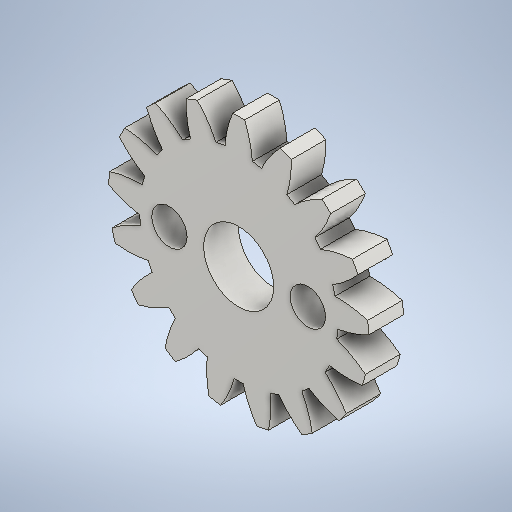
# Autodesk Inventor part: 平歯車1
Saved by Autodesk Inventor 2025.1 (Build 291241000, 241)
## iProperties
CustomPartVersion: 1
Created: 2025-05-06
Part Number: 平歯車1
Material: Steel
Document SubType Name: Modeling
Designer: yuki0520
Categories: <?xml version="1.0" encoding="UTF-16"?> <MemberInstance><Categories><FamilyTemplate><FamilyTemplateParameter ValueType="xs:double" Id="1" ObjectReferenceKey="da_z" ObjectType="kUserParameterObject"/><FamilyTemplateParameter ValueType="xs:double" Id="2" ObjectReferenceKey="da_b" ObjectType="kUserParameterObject"/><FamilyTemplateParameter ValueType="xs:double" Id="3" ObjectReferenceKey="da_beta" ObjectType="kUserParameterObject"/><FamilyTemplateParameter ValueType="xs:double" Id="4" ObjectReferenceKey="da_da" ObjectType="kUserParameterObject"/><FamilyTemplateParameter ValueType="xs:double" Id="5" ObjectReferenceKey="da_aw" ObjectType="kUserParameterObject"/><FamilyTemplateParameter ValueType="xs:string" Id="6" ObjectReferenceKey="EAIAABAAAACIAQAAAAAAAIAAAAAAAAAA" ObjectType="83910656" SubObjectId="SurfaceGeometry"/></FamilyTemplate><ParamToTemplateMap><ParamToTemplate CategoryParameter="//CategoryParameter[@InternalName='046C89C9-8512-4d59-83FE-43B91F4F132A']" TemplateParameter="1"/><ParamToTemplate CategoryParameter="//CategoryParameter[@InternalName='2552DF32-E462-4b46-AEBF-C6C7768E72AC']" TemplateParameter="2"/><ParamToTemplate CategoryParameter="//CategoryParameter[@InternalName='C9EE641D-15FC-4fae-A226-E94C4372FDD7']" TemplateParameter="3"/><ParamToTemplate><ParamToTemplate CategoryParameter="//CategoryParameter[@InternalName='00B6519A-459B-49c7-AD84-2E56D39A5744']" ConstantValue="-0.100000"/></ParamToTemplate><ParamToTemplate><ParamToTemplate CategoryParameter="//CategoryParameter[@InternalName='04B31F0E-C7A6-4894-AA32-9629BEFACF47']" ConstantValue="1.000000"/></ParamToTemplate><ParamToTemplate><ParamToTemplate CategoryParameter="//CategoryParameter[@InternalName='43CBEC2E-7847-49e7-A936-2F7889FCB2D9']" ConstantValue="0.250000"/></ParamToTemplate><ParamToTemplate><ParamToTemplate CategoryParameter="//CategoryParameter[@InternalName='B1EFC894-105D-4ebd-86BF-FA20ED196853']" ConstantValue="0.350000"/></ParamToTemplate><ParamToTemplate><ParamToTemplate CategoryParameter="//CategoryParameter[@InternalName='51175063-3D10-4879-93E8-6246FE8B403D']" ConstantValue="2060000000.000000"/></ParamToTemplate><ParamToTemplate><ParamToTemplate CategoryParameter="//CategoryParameter[@InternalName='A3A52E27-4454-46a9-B0BD-C932399B70AF']" ConstantValue="0.300000"/></ParamToTemplate><ParamToTemplate><ParamToTemplate CategoryParameter="//CategoryParameter[@InternalName='91B76062-C214-41d9-B1B9-14D2AB99603D']" ConstantValue="0.200000"/></ParamToTemplate><ParamToTemplate><ParamToTemplate CategoryParameter="//CategoryParameter[@InternalName='374E806E-8B8A-4dda-A9AA-1039D6500AD2']" ConstantValue="5.000000"/></ParamToTemplate><ParamToTemplate><ParamToTemplate CategoryParameter="//CategoryParameter[@InternalName='2D373A89-B862-43d6-8D0B-0CBF12AB9F6C']" ConstantValue="0.349066"/></ParamToTemplate><ParamToTemplate CategoryParameter="//CategoryParameter[@InternalName='37777632-D6A2-4fac-9D53-DB8ACD95C989']" TemplateParameter="4"/><ParamToTemplate CategoryParameter="//CategoryParameter[@InternalName='FD1017F1-B727-4f7e-9707-0F86F1FF9423']" TemplateParameter="5"/><ParamToTemplate><ParamToTemplate CategoryParameter="//CategoryParameter[@InternalName='9E1B4470-B2D3-4ff1-B813-535BB4CDF51A']" ConstantValue="3520000.000000"/></ParamToTemplate><ParamToTemplate><ParamToTemplate CategoryParameter="//CategoryParameter[@InternalName='F8452263-BFF6-458c-9FB1-07C4B99E95CD']" ConstantValue="11400000.000000"/></ParamToTemplate><ParamToTemplate><ParamToTemplate CategoryParameter="//CategoryParameter[@InternalName='3E3BB259-FD49-497f-8171-6EBC954A3479']" ConstantValue="2.000000"/></ParamToTemplate><ParamToTemplate CategoryParameter="//CategoryParameter[@InternalName='27C3BAF2-7550-4e4b-AE2C-0DB134B7D9B7']" TemplateParameter="6"/></ParamToTemplateMap><Category DisplayName="Gear" InternalName="DC85795E-93AB-48d5-8EEE-5A27447B64BD" Mnemonic="Gear"><CategoryParameter DisplayName="z" InternalName="046C89C9-8512-4d59-83FE-43B91F4F132A" Mnemonic="z"/><CategoryParameter DisplayName="b" InternalName="2552DF32-E462-4b46-AEBF-C6C7768E72AC" Mnemonic="b"/><CategoryParameter DisplayName="||b|" InternalName="C9EE641D-15FC-4fae-A226-E94C4372FDD7" Mnemonic="beta"/><CategoryParameter DisplayName="x" InternalName="00B6519A-459B-49c7-AD84-2E56D39A5744" Mnemonic="x"/><CategoryParameter DisplayName="a*" InternalName="04B31F0E-C7A6-4894-AA32-9629BEFACF47" Mnemonic="a"/><CategoryParameter DisplayName="c*" InternalName="43CBEC2E-7847-49e7-A936-2F7889FCB2D9" Mnemonic="c"/><CategoryParameter DisplayName="r|.f|*" InternalName="B1EFC894-105D-4ebd-86BF-FA20ED196853" Mnemonic="rf"/><CategoryParameter DisplayName="E" InternalName="51175063-3D10-4879-93E8-6246FE8B403D" Mnemonic="E"/><CategoryParameter DisplayName="||m|" InternalName="A3A52E27-4454-46a9-B0BD-C932399B70AF" Mnemonic="mi"/><Category DisplayName="SpurGear" InternalName="26C5A22E-A91E-4dfd-A3B3-23CCAFAE1764" Mnemonic="SpurGear"><CategoryParameter DisplayName="m" InternalName="91B76062-C214-41d9-B1B9-14D2AB99603D" Mnemonic="m"/><CategoryParameter DisplayName="P" InternalName="374E806E-8B8A-4dda-A9AA-1039D6500AD2" Mnemonic="PP"/><CategoryParameter DisplayName="||a|" InternalName="2D373A89-B862-43d6-8D0B-0CBF12AB9F6C" Mnemonic="alpha"/><CategoryParameter DisplayName="d|.a|" InternalName="37777632-D6A2-4fac-9D53-DB8ACD95C989" Mnemonic="da"/><CategoryParameter DisplayName="a|.w|" InternalName="FD1017F1-B727-4f7e-9707-0F86F1FF9423" Mnemonic="aw"/><CategoryParameter DisplayName="||s||.Flim|" InternalName="9E1B4470-B2D3-4ff1-B813-535BB4CDF51A" Mnemonic="sFlim"/><CategoryParameter DisplayName="||s||.Hlim|" InternalName="F8452263-BFF6-458c-9FB1-07C4B99E95CD" Mnemonic="sHlim"/><CategoryParameter DisplayName="タイプ" InternalName="3E3BB259-FD49-497f-8171-6EBC954A3479" Mnemonic="type"/><CategoryParameter DisplayName="PitchDiameter" InternalName="27C3BAF2-7550-4e4b-AE2C-0DB134B7D9B7" Mnemonic="IDS_PITCHDIAM"/></Category></Category></Categories></MemberInstance>
Density: 1 g/cm^3
Appearance: Steel
Author: yuki0520
Autodesk Inventor part; units mm, degrees
sketch "Sketch1" plane through (0, 0, 0) normal (0, 0, 1) x (1, 0, 0)
  circle A0 centre (0, 0) radius 18.8
  dimension "d0" = 37.6
  constraints: 1 centre point
  measures "d0" diameter of A0
extrude "Extrusion1" add sketch "Sketch1" along normal blind 5
ref_plane "Work Plane2" through (0, 0, 2.5) normal (0, 0, 1) x (1, 0, 0)
sketch "Sketch2" plane through (0, 0, 0) normal (0, 0, -1) x (-1, 0, 0)
  circle A0 centre (0, 0) radius 18.8 projected
  circle A1 centre (0, 0) radius 17
  dimension "d3" = 34
  constraints: 1 centre point, 1 coincident
  measures "d3" diameter of A1
surface extrude "ピッチ円直径" sketch "Sketch2" against normal through all shown no curves A1
ref_plane "Work Plane8" through (0, 0, 0) normal (0.9829731, 0.1837495, 0) x (0, 0, 1)
ref_plane "Work Plane9" through (0, 0, 0) normal (1, 0, 0) x (0, 1, 0)
spur gear teeth "平歯車" teeth 17 pitch diameter 34 tip diameter 37.6 root diameter 28.6 face width 5 start plane through (0, 0, 0) normal (0, 0, -1) x (-1, 0, 0)
sketch "スケッチ3" plane through (0, 0, 5) normal (0, 0, 1) x (1, 0, 0)
  arc A0 (-5.9745, 17.8254) -> (-7.5937, 17.1981) centre (0, 0) ccw projected
  arc A1 (-7.5937, 17.1981) -> (-6.9584, 12.4928) centre (7.6342, 16.8585) ccw projected
  arc A2 (-6.9584, 12.4928) -> (-8.0815, 11.7975) centre (0, 0) ccw projected
  arc A3 (-8.0815, 11.7975) -> (-12.0103, 14.4635) centre (-18.494, 0.6806) ccw projected
  arc A4 (-12.0103, 14.4635) -> (-13.2936, 13.2936) centre (0, 0) ccw projected
  arc A5 (-13.2936, 13.2936) -> (-11.0015, 9.1355) centre (1.0287, 18.4779) ccw projected
  arc A6 (-11.0015, 9.1355) -> (-11.7975, 8.0815) centre (0, 0) ccw projected
  arc A7 (-11.7975, 8.0815) -> (-16.4241, 9.1482) centre (-17.491, -6.0461) ccw projected
  arc A8 (-16.4241, 9.1482) -> (-17.1981, 7.5937) centre (0, 0) ccw projected
  arc A9 (-17.1981, 7.5937) -> (-13.5587, 4.5444) centre (-5.7158, 17.6017) ccw projected
  arc A10 (-13.5587, 4.5444) -> (-13.9202, 3.274) centre (0, 0) ccw projected
  arc A11 (-13.9202, 3.274) -> (-18.6197, 2.5973) centre (-14.1258, -11.9563) ccw projected
  arc A12 (-18.6197, 2.5973) -> (-18.7799, 0.8682) centre (0, 0) ccw projected
  arc A13 (-18.7799, 0.8682) -> (-14.2847, -0.6604) centre (-11.6883, 14.3483) ccw projected
  arc A14 (-14.2847, -0.6604) -> (-14.1629, -1.9756) centre (0, 0) ccw projected
  arc A15 (-14.1629, -1.9756) -> (-18.3006, -4.3043) centre (-8.8528, -16.2517) ccw projected
  arc A16 (-18.3006, -4.3043) -> (-17.8254, -5.9745) centre (0, 0) ccw projected
  arc A17 (-17.8254, -5.9745) -> (-13.0816, -5.7761) centre (-16.0822, 9.1571) ccw projected
  arc A18 (-13.0816, -5.7761) -> (-12.4928, -6.9584) centre (0, 0) ccw projected
  arc A19 (-12.4928, -6.9584) -> (-15.51, -10.6246) centre (-2.3841, -18.3523) ccw projected
  arc A20 (-15.51, -10.6246) -> (-14.4635, -12.0103) centre (0, 0) ccw projected
  arc A21 (-14.4635, -12.0103) -> (-10.1116, -10.1116) centre (-18.3041, 2.7292) ccw projected
  arc A22 (-10.1116, -10.1116) -> (-9.1355, -11.0015) centre (0, 0) ccw projected
  arc A23 (-9.1355, -11.0015) -> (-10.6246, -15.51) centre (4.4065, -17.9742) ccw projected
  arc A24 (-10.6246, -15.51) -> (-9.1482, -16.4241) centre (0, 0) ccw projected
  arc A25 (-9.1482, -16.4241) -> (-5.7761, -13.0816) centre (-18.054, -4.0673) ccw projected
  arc A26 (-5.7761, -13.0816) -> (-4.5444, -13.5587) centre (0, 0) ccw projected
  arc A27 (-4.5444, -13.5587) -> (-4.3043, -18.3006) centre (10.6019, -15.1687) ccw projected
  arc A28 (-4.3043, -18.3006) -> (-2.5973, -18.6197) centre (0, 0) ccw projected
  arc A29 (-2.5973, -18.6197) -> (-0.6604, -14.2847) centre (-15.3656, -10.3145) ccw projected
  arc A30 (-0.6604, -14.2847) -> (0.6604, -14.2847) centre (0, 0) ccw projected
  arc A31 (0.6604, -14.2847) -> (2.5973, -18.6197) centre (15.3656, -10.3145) ccw projected
  arc A32 (2.5973, -18.6197) -> (4.3043, -18.3006) centre (0, 0) ccw projected
  arc A33 (4.3043, -18.3006) -> (4.5444, -13.5587) centre (-10.6019, -15.1687) ccw projected
  arc A34 (4.5444, -13.5587) -> (5.7761, -13.0816) centre (0, 0) ccw projected
  arc A35 (5.7761, -13.0816) -> (9.1482, -16.4241) centre (18.054, -4.0673) ccw projected
  arc A36 (9.1482, -16.4241) -> (10.6246, -15.51) centre (0, 0) ccw projected
  arc A37 (10.6246, -15.51) -> (9.1355, -11.0015) centre (-4.4065, -17.9742) ccw projected
  arc A38 (9.1355, -11.0015) -> (10.1116, -10.1116) centre (0, 0) ccw projected
  arc A39 (10.1116, -10.1116) -> (14.4635, -12.0103) centre (18.3041, 2.7292) ccw projected
  arc A40 (14.4635, -12.0103) -> (15.51, -10.6246) centre (0, 0) ccw projected
  arc A41 (15.51, -10.6246) -> (12.4928, -6.9584) centre (2.3841, -18.3523) ccw projected
  arc A42 (12.4928, -6.9584) -> (13.0816, -5.7761) centre (0, 0) ccw projected
  arc A43 (13.0816, -5.7761) -> (17.8254, -5.9745) centre (16.0822, 9.1571) ccw projected
  arc A44 (17.8254, -5.9745) -> (18.3006, -4.3043) centre (0, 0) ccw projected
  arc A45 (18.3006, -4.3043) -> (14.1629, -1.9756) centre (8.8528, -16.2517) ccw projected
  arc A46 (14.1629, -1.9756) -> (14.2847, -0.6604) centre (0, 0) ccw projected
  arc A47 (14.2847, -0.6604) -> (18.7799, 0.8682) centre (11.6883, 14.3483) ccw projected
  arc A48 (18.7799, 0.8682) -> (18.6197, 2.5973) centre (0, 0) ccw projected
  arc A49 (18.6197, 2.5973) -> (13.9202, 3.274) centre (14.1258, -11.9563) ccw projected
  arc A50 (13.9202, 3.274) -> (13.5587, 4.5444) centre (0, 0) ccw projected
  arc A51 (13.5587, 4.5444) -> (17.1981, 7.5937) centre (5.7158, 17.6017) ccw projected
  arc A52 (17.1981, 7.5937) -> (16.4241, 9.1482) centre (0, 0) ccw projected
  arc A53 (16.4241, 9.1482) -> (11.7975, 8.0815) centre (17.491, -6.0461) ccw projected
  arc A54 (11.7975, 8.0815) -> (11.0015, 9.1355) centre (0, 0) ccw projected
  arc A55 (11.0015, 9.1355) -> (13.2936, 13.2936) centre (-1.0287, 18.4779) ccw projected
  arc A56 (13.2936, 13.2936) -> (12.0103, 14.4635) centre (0, 0) ccw projected
  arc A57 (12.0103, 14.4635) -> (8.0815, 11.7975) centre (18.494, 0.6806) ccw projected
  arc A58 (8.0815, 11.7975) -> (6.9584, 12.4928) centre (0, 0) ccw projected
  arc A59 (6.9584, 12.4928) -> (7.5937, 17.1981) centre (-7.6342, 16.8585) ccw projected
  arc A60 (7.5937, 17.1981) -> (5.9745, 17.8254) centre (0, 0) ccw projected
  arc A61 (5.9745, 17.8254) -> (3.274, 13.9202) centre (16.9992, 7.3155) ccw projected
  arc A62 (3.274, 13.9202) -> (1.9756, 14.1629) centre (0, 0) ccw projected
  arc A63 (1.9756, 14.1629) -> (0.8682, 18.7799) centre (-13.2087, 12.9623) ccw projected
  arc A64 (0.8682, 18.7799) -> (-0.8682, 18.7799) centre (0, 0) ccw projected
  arc A65 (-0.8682, 18.7799) -> (-1.9756, 14.1629) centre (13.2087, 12.9623) ccw projected
  arc A66 (-1.9756, 14.1629) -> (-3.274, 13.9202) centre (0, 0) ccw projected
  arc A67 (-3.274, 13.9202) -> (-5.9745, 17.8254) centre (-16.9992, 7.3155) ccw projected
  circle A68 centre (0, 0) radius 5.05
  circle A69 centre (0, 0) radius 10
  line L0 (-10, 0) -> (10, 0)
  circle A70 centre (10, 0) radius 2.55
  circle A71 centre (-10, 0) radius 2.55
  arc A72 (8.0815, 11.7975) -> (6.9584, 12.4928) centre (0, 0) ccw projected
  dimension "d49" = 10.1
  dimension "d50" = 20
  dimension "d51" = 5.1
  dimension "d52" = 5.1
  dimension "d55" = 14.3
  constraints: 4 centre point, 3 coincident, 2 end point, 2 midpoint, 2 point on circle, 1 concentric, 1 horizontal
  measures "d49" diameter of A68
  measures "d50" diameter of A69
  measures "d51" diameter of A70
  measures "d52" diameter of A71
  measures "d55" radius of A62
extrude "押し出し2" cut sketch "スケッチ3" against normal blind 10 contours L0 A68 | A68 L0 | A70 A69 L0 | L0 A69 A70 | A71 A69 L0 | L0 A69 A71 | A69 A70 | A69 A71
equation "\"d0\" = da_da"
equation "\"d1\" = da_b"
equation "\"d3\" = da_d"
equation "\"d16\" = da_aw"
equation "\"d43\" = da_aw"
equation "\"d46\" = da_aw"
equation "\"da_da\" = 37.6"
equation "\"da_b\" = 5"
equation "\"da_d\" = 34"
equation "\"da_aw\" = 34"
body "Solid1"
body "Srf1"
